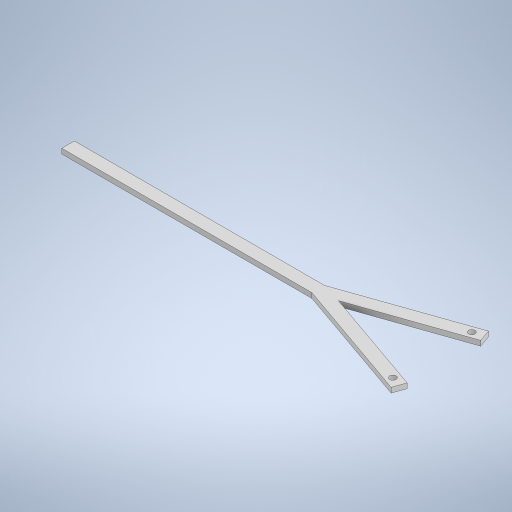
# Autodesk Inventor part: connector
Saved by Autodesk Inventor 2024 (Build 280153000, 153)
## iProperties
Created: 2024-10-22
Part Number: connector
Material: Generic
Document SubType Name: Modeling
Designer: kamil
Density: 1 g/cm^3
Appearance: Default
Author: kamil
Autodesk Inventor part; units mm, degrees
ref_plane "YZ Plane" through (0, 0, 0) normal (1, 0, 0) x (0, 1, 0)
ref_plane "XZ Plane" through (0, 0, 0) normal (0, 1, 0) x (-1, 0, 0)
ref_plane "XY Plane" through (0, 0, 0) normal (0, 0, 1) x (1, 0, 0)
sketch "Sketch1" plane through (0, 0, 0) normal (0, 1, 0) x (-1, 0, 0)
  line L0 (-11.9073, -0.0524) -> (-8.2127, -0.0524) construction
  line L1 (0, 0) -> (-37.2003, 0) construction
  line L2 (-11.9073, -0.0524) -> (-8.256, -0.0524) construction
  line L3 (0, 2.4476) -> (0, 12.311) construction
  line L4 (-25, -2.5) -> (75, -2.5)
  line L5 (75, -2.5) -> (75, 2.5)
  line L6 (75, 2.5) -> (-25, 2.5)
  line L7 (-25, 2.5) -> (-25, -2.5)
  line L8 (-25, 0) -> (75, 0) construction
  line L9 (25, -2.5) -> (25, 2.5) construction
  circle A0 centre (-70, 15.69) radius 1.3
  circle A1 centre (-70, -15.69) radius 1.3
  line L10 (-25.8231, -2.3606) -> (-24.1769, 2.3606)
  line L11 (-24.1769, 2.3606) -> (-72.9539, 19.3675)
  line L12 (-72.9539, 19.3675) -> (-74.6001, 14.6463)
  line L13 (-74.6001, 14.6463) -> (-25.8231, -2.3606)
  line L14 (-73.777, 17.0069) -> (-25, 0)
  line L15 (-25.8231, 2.3606) -> (-24.1769, -2.3606)
  line L16 (-24.1769, -2.3606) -> (-72.9539, -19.3675)
  line L17 (-72.9539, -19.3675) -> (-74.6001, -14.6463)
  line L18 (-74.6001, -14.6463) -> (-25.8231, 2.3606)
  line L19 (-73.777, -17.0069) -> (-25, 0)
  point P0 (-24.5767, 2.5)
  point P1 (-32.5935, 0)
  point P2 (-24.5767, -2.5)
  dimension "d10" = 5
  dimension "d12" = 100
  dimension "d13" = 50
  dimension "d18" = 2.6
  dimension "d19" = 15.69
  dimension "d21" = 70
  dimension "d24" = 5
  dimension "d25" = 4
  dimension "d26" = 75
  constraints: 40 end point, 6 midpoint, 6 symmetric about line, 4 horizontal, 4 parallel, 2 centre point, 2 perpendicular, 1 collinear, 1 point on line, 1 other
  measures "d10" distance of L4.end L5.end
  measures "d12" distance of L8.end L8.start
  measures "d13" distance between parallel lines of L5 L9
  measures "d18" diameter of A0
  measures "d19" distance from line of L1 A0.centre
  measures "d21" horizontal distance of L1.start A0.centre
  measures "d24" distance of L11.end L12.end
  measures "d25" distance from line of L12 A0.centre
  measures "d26" distance from line of L1.start L5
extrude "Extrusion1" add sketch "Sketch1" along normal blind 2 contours L7 L15 L16 L4 | L4 L16 L17 L19 A1 L13 L10 L7 | L16 L15 L10 L11 L6 L5 L4 | L15 L18 L14 A0 L12 L11 L6 L7 | L7 L6 L11 L10 | L19 L13 L18 L14 | L14 L18 L15 | L10 L13 L19 | L18 L13 L12 L14 A0 | L19 A1 L17 L18 L13
body "Solid1"
